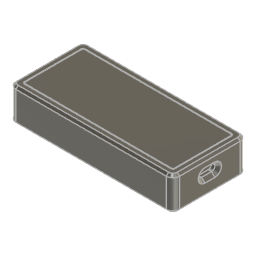
Auto seat warmer (Autodesk Fusion 360 design; units mm, degrees)
Autodesk Fusion 360 part; units mm, degrees
note: some values were not read from the file. Set by a fixed rule: which face or edge a step refers to.
sketch "Sketch1" plane through (0, 0, 0) normal (0, 0, 1) x (1, 0, 0)
  line L0 (0, 0) -> (45.2, 0)
  line L1 (45.2, 0) -> (45.2, 18.2)
  line L2 (45.2, 18.2) -> (0, 18.2)
  line L3 (0, 18.2) -> (0, 0)
  line L4 (-2, 20.2) -> (47.2, 20.2)
  line L5 (47.2, 20.2) -> (47.2, -2)
  line L6 (47.2, -2) -> (-2, -2)
  line L7 (-2, -2) -> (-2, 20.2)
  dimension "d1" = 45.2
  dimension "d2" = 18.2
  dimension "d3" = 2
  dimension "d4" = 2
  dimension "d5" = 2
  dimension "d6" = 2
  constraint horizontal L0
  constraint vertical L1
  constraint horizontal L2
  constraint vertical L3
  constraint coincident L0.start L3.end
  constraint horizontal L4
  constraint vertical L5
  constraint horizontal L6
  constraint vertical L7
  measures "d1" distance of L0.start L0.end
  measures "d2" distance of L0.start L2.end
  measures "d3" distance of L3 L7
  measures "d4" distance of L2 L4
  measures "d5" distance of L1 L5
  measures "d6" distance of L0 L6
extrude "Extrude1" add sketch "Sketch1" along normal blind 2 contours L0 L1 L2 L3 makes body 1 in component "Component"
extrude "Extrude2" add sketch "Sketch1" along normal blind 10 bodies 1 in component "Component"
extrude "Extrude1'" add sketch "Sketch1" against normal blind 3 from surface at 10 separate body contours L0 L1 L2 L3 makes body 2 in component "Component'"
sketch "Sketch2" plane through (0, 0, 0) normal (0, 1, 0) x (-1, 0, 0)
  line L0 (-45.2, 2) -> (0, 2)
  line L1 (0, 2) -> (0, 10)
  line L2 (0, 10) -> (-45.2, 10)
  line L3 (-45.2, 10) -> (-45.2, 2)
  line L4 (-22.6, 2) -> (-22.6, 13) construction
  circle A0 centre (-40.2, 8) radius 1
  circle A1 centre (-5, 8) radius 1
  circle A2 centre (-5, 8) radius 0.9
  circle A3 centre (-40.2, 8) radius 0.9
  dimension "d18" = 2
  dimension "d19" = 2
  dimension "d20" = 5
  dimension "d47" = -0.1
  constraint midpoint L0 L4.start
  constraint perpendicular L2 L4
  constraint symmetric L4 A0 A1
  constraint symmetric L4 A2 A3
  measures "d18" diameter of A0
  measures "d19" distance of L2 A0.centre
  measures "d20" distance of L3 A0.centre
extrude "Extrude3" cut sketch "Sketch2" against normal blind 1 contours A0 | A1 | A2 | A3 bodies 1 in component "Component"
extrude "Extrude4" cut sketch "Sketch2" along normal blind 1 from surface at 18.2 contours A0 | A1 | A2 | A3 bodies 1 in component "Component"
fillet "Fillet1" radius 1 4 edges at (5.9323, 19.2, 7.6384) (41.1323, 19.2, 7.6384) (5.9323, -1, 8.3616) (41.1323, -1, 8.3616) on bodies 1 in component "Component"
move_face "OffsetFaces1" offset -0.15 4 faces at (15.0667, 0, 9) (0, 12.1333, 9) (30.1333, 18.2, 9) (45.2, 6.0667, 9) on bodies 2 in component "Component'"
extrude "Extrude2'" add sketch "Sketch2" against normal blind 0.8 from surface at 0.15 contours A2 | A3 bodies 2 in component "Component'"
extrude "Extrude3'" add sketch "Sketch2" along normal blind 0.8 from surface at 18.05 contours A2 | A3 bodies 2 in component "Component'"
fillet "Fillet1'" radius 0.8 4 faces at (40.2224, 18.85, 8.2858) (4.7133, 18.85, 7.9116) (40.2224, -0.65, 8.2858) (4.7133, -0.65, 7.9116) on bodies 2 in component "Component'"
sketch "Sketch3" plane through (0, 0, 0) normal (1, 0, 0) x (0, 1, 0)
  line L0 (0, 2) -> (18.2, 2)
  line L1 (18.2, 2) -> (18.2, 10)
  line L2 (18.2, 10) -> (0, 10)
  line L3 (0, 10) -> (0, 2)
  line L4 (9.1, 2) -> (9.1, 6.8) construction
  line L5 (6.1, 6.8) -> (12.1, 6.8) construction
  line L6 (4.7, 5.4) -> (4.7, 5) construction
  line L7 (6.1, 3.6) -> (12.1, 3.6) construction
  line L8 (13.5, 5.4) -> (13.5, 5) construction
  arc A0 (6.1, 6.8) -> (4.7, 5.4) centre (6.1, 5.4) ccw construction
  arc A1 (13.5, 5.4) -> (12.1, 6.8) centre (12.1, 5.4) ccw construction
  arc A2 (12.1, 3.6) -> (13.5, 5) centre (12.1, 5) ccw construction
  arc A3 (4.7, 5) -> (6.1, 3.6) centre (6.1, 5) ccw construction
  arc A4 (13.8, 5.4) -> (12.1, 7.1) centre (12.1, 5.4) ccw
  line L9 (6.1, 7.1) -> (12.1, 7.1)
  arc A5 (6.1, 7.1) -> (4.4, 5.4) centre (6.1, 5.4) ccw
  line L10 (4.4, 5.4) -> (4.4, 5)
  arc A6 (4.4, 5) -> (6.1, 3.3) centre (6.1, 5) ccw
  line L11 (6.1, 3.3) -> (12.1, 3.3)
  arc A7 (12.1, 3.3) -> (13.8, 5) centre (12.1, 5) ccw
  line L12 (13.8, 5.4) -> (13.8, 5)
  dimension "d36" = 3.2
  dimension "d37" = 1.6
  dimension "d38" = 8.8
  dimension "d39" = 1.4
  dimension "d40" = -0.3
  constraint midpoint L0 L4.start
  constraint perpendicular L2 L4
  constraint perpendicular L4 L5
  constraint perpendicular L6 L7
  constraint perpendicular L0 L8
  constraint equal L5 L7
  constraint midpoint L4.end L5
  constraint tangent L6 A0
  constraint tangent L8 A1
  constraint tangent L8 A2
  constraint tangent L6 A3
  constraint equal A0 A1
  constraint equal A0 A3
  constraint equal A0 A2
  constraint tangent L5 A0
  constraint tangent L7 A3
  constraint tangent L7 A2
  measures "d36" distance of L5 L7
  measures "d37" distance of L0 L7
  measures "d38" distance of L6 L8
  measures "d39" radius of A0
extrude "Extrude5" cut sketch "Sketch3" against normal blind 2 contours A4 L9 A5 L10 A6 L11 A7 L12 bodies 1 in component "Component"
fillet "Fillet2" radius 2 4 edges at (-2, -2, 5) (47.2, -2, 5) (47.2, 20.2, 5) (-2, 20.2, 5) on bodies 1 in component "Component"
chamfer "Chamfer1" distance 0.7 angle 45 8 edges at (-2, 9.1, 10) (-1.4142, -1.4142, 10) (22.6, -2, 10) (46.6142, -1.4142, 10) (47.2, 9.1, 10) (46.6142, 19.6142, 10) (22.6, 20.2, 10) (-1.4142, 19.6142, 10) 1 faces at (15.0667, 5.4, 0) on bodies 1 in component "Component"
sketch "Sketch4" plane through (47.2, 0, 0) normal (1, 0, 0) x (0, 1, 0)
  line L0 (0, 0.7) -> (18.2, 0.7)
  line L1 (18.2, 0.7) -> (18.2, 9.3)
  line L2 (18.2, 9.3) -> (0, 9.3)
  line L3 (0, 9.3) -> (0, 0.7)
  line L4 (7.6, 4.7) -> (10.6, 4.7)
  arc A0 (10.6, 4.7) -> (10.6, 6.7) centre (10.6, 5.7) ccw
  line L5 (10.6, 6.7) -> (7.6, 6.7)
  arc A1 (7.6, 6.7) -> (7.6, 4.7) centre (7.6, 5.7) ccw
  line L6 (7.6, 5.7) -> (10.6, 5.7) construction
  line L7 (9.1, 0.7) -> (9.1, 5.7) construction
  dimension "d50" = 2
  dimension "d51" = 3
  dimension "d52" = 4
  constraint tangent L4 A0
  constraint tangent A0 L5
  constraint parallel L4 L5
  constraint tangent L5 A1
  constraint tangent L4 A1
  constraint horizontal L6
  constraint midpoint L0 L7.start
  constraint perpendicular L0 L7
  constraint midpoint L6 L7.end
  measures "d50" distance of L4 L5
  measures "d51" distance of A1.centre A0.centre
  measures "d52" distance of L0 L4
extrude "Extrude6" cut sketch "Sketch4" against normal blind 2 contours L4 A0 L5 A1 bodies 1 in component "Component"
chamfer "Chamfer2" distance 1 angle 45 12 edges at (-2, 13.3021, 3.7979) (-2, 13.8, 5.2) (-2, 13.3021, 6.6021) (-2, 9.1, 7.1) (-2, 4.8979, 6.6021) (-2, 4.4, 5.2) (-2, 4.8979, 3.7979) (-2, 9.1, 3.3) (47.2, 9.1, 4.7) (47.2, 6.6, 5.7) (47.2, 9.1, 6.7) (47.2, 11.6, 5.7) on bodies 1 in component "Component"
fillet "Fillet2'" radius 0.5 4 edges at (0.15, 0.15, 8.5) (0.15, 18.05, 8.5) (45.05, 18.05, 8.5) (45.05, 0.15, 8.5) on bodies 2 in component "Component'"
fillet "Fillet3" radius 0.5 4 edges at (0, 0, 6) (0, 18.2, 6) (45.2, 18.2, 6) (45.2, 0, 6) on bodies 1 in component "Component"
component "Component" placed x (1, 0, 0) y (0, 1, 0) z (0, 0, 1) at (0, 0, 0)
component "Component'" placed x (1, 0, 0) y (0, 1, 0) z (0, 0, 1) at (0, 0, 0)
equation "d4 = d3"
equation "d5 = d3"
equation "d6 = d3"
